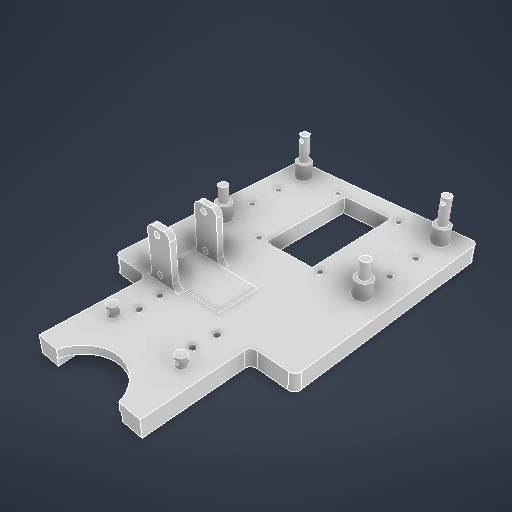
# Autodesk Inventor part: Lower_Chassis
Saved by Autodesk Inventor 2025 (Build 290162000, 162)
## iProperties
Created: 2024-06-03
Part Number: Lower_Chassis
Material: Generic
Document SubType Name: Modeling
Designer: Garfieldcmix
Density: 1 g/cm^3
Appearance: Default
Author: Garfieldcmix
Autodesk Inventor part; units mm, degrees
ref_plane "YZ Plane" through (0, 0, 0) normal (1, 0, 0) x (0, 1, 0)
ref_plane "XZ Plane" through (0, 0, 0) normal (0, 1, 0) x (-1, 0, 0)
derived "Car_Plan.ipt"
sketch "Car_Sketch" plane through (0, 0, 0) normal (0, 1, 0) x (-1, 0, 0)
  line L0 (0, 0) -> (94, 0)
  line L1 (0, 0) -> (0, 105)
  line L2 (94, 0) -> (94, 105)
  line L3 (0, 105) -> (20, 105)
  line L4 (20, 105) -> (20, 190)
  line L5 (20, 190) -> (74, 190)
  line L6 (74, 190) -> (74, 105)
  line L7 (74, 105) -> (94, 105)
  line L8 (-5, 68) -> (-5, 0)
  line L9 (-5, 0) -> (-32, 0)
  line L10 (-32, 0) -> (-32, 68)
  line L11 (-32, 68) -> (-5, 68)
  line L12 (47, 190) -> (47, 0) construction
  line L13 (126, 68) -> (99, 68)
  line L14 (99, 68) -> (99, 0)
  line L15 (126, 0) -> (126, 68)
  line L16 (99, 0) -> (126, 0)
  line L17 (-5, 34) -> (99, 34) construction
  line L18 (0, 95) -> (94, 95) construction
  line L19 (-5, 190) -> (-32, 190)
  line L20 (-32, 122) -> (-5, 122)
  line L21 (-32, 190) -> (-32, 122)
  line L22 (-5, 122) -> (-5, 190)
  line L23 (-5, 156) -> (99, 156) construction
  line L24 (126, 122) -> (99, 122)
  line L25 (126, 190) -> (126, 122)
  line L26 (99, 190) -> (126, 190)
  line L27 (99, 122) -> (99, 190)
  line L28 (0, 156) -> (47, 34) construction
  line L29 (94, 156) -> (47, 34) construction
  line L30 (0, 156) -> (-174.2341, 34) construction
  line L31 (-5, 34) -> (-174.2341, 34) construction
  line L32 (8.9873, 132.6713) -> (47, 142.55) construction
  line L33 (85.0127, 132.6713) -> (47, 142.55) construction
derived "Front_Bridge.ipt"
sketch "Front_Bridge_Base" plane through (0, 0, 0) normal (0, 1, 0) x (-1, 0, 0)
  circle A0 centre (0, 156) radius 1.5
  circle A1 centre (94, 156) radius 1.5
  line L0 (-5, 161) -> (-5, 151)
  line L1 (-5, 151) -> (29.5, 151)
  line L2 (99, 151) -> (99, 161)
  line L3 (99, 161) -> (90, 161)
  line L4 (4, 161) -> (22, 190)
  line L5 (22, 190) -> (72, 190)
  line L6 (72, 190) -> (90, 161)
  line L7 (0, 156) -> (94, 156) construction
  line L8 (4, 161) -> (-5, 161)
  line L9 (40.95, 172.3) -> (53.05, 172.3)
  line L10 (53.05, 172.3) -> (53.05, 149.9)
  line L11 (53.05, 149.9) -> (40.95, 149.9)
  line L12 (40.95, 149.9) -> (40.95, 172.3)
  line L13 (47, 156) -> (47, 149.9) construction
  line L14 (32, 151) -> (37, 144)
  line L15 (37, 144) -> (57, 144)
  line L16 (57, 144) -> (62, 151)
  line L17 (47, 156) -> (47, 144) construction
  line L18 (32, 151) -> (62, 151)
  line L19 (62, 151) -> (64.5, 151)
  line L20 (29.5, 151) -> (24.5, 102)
  line L21 (24.5, 102) -> (69.5, 102)
  line L22 (69.5, 102) -> (64.5, 151)
  line L23 (64.5, 151) -> (99, 151)
  line L24 (29.5, 151) -> (32, 151)
  line L25 (4, 161) -> (4, 151)
  line L26 (90, 161) -> (90, 151)
  circle A2 centre (32, 109) radius 1.5
  circle A3 centre (33, 119) radius 1.5
  line L27 (47, 156) -> (47, 102) construction
  circle A4 centre (61, 119) radius 1.5
  circle A5 centre (62, 109) radius 1.5
  line L28 (9, 169.0556) -> (9, 151)
  line L29 (84.8333, 151) -> (84.5992, 150.8961)
  line L30 (85, 169.0556) -> (85, 151)
  line L31 (26, 190) -> (26, 151)
  line L32 (68, 190) -> (68, 151)
  circle A6 centre (17, 157) radius 1.5
  circle A7 centre (17, 169) radius 1.5
  circle A8 centre (77, 157) radius 1.5
  circle A9 centre (77, 169) radius 1.5
  line L33 (37.95, 162.3) -> (33.95, 162.3)
  line L34 (33.95, 162.3) -> (33.95, 172.3)
  line L35 (33.95, 172.3) -> (37.95, 172.3)
  line L36 (37.95, 172.3) -> (37.95, 162.3)
  circle A10 centre (47, 156) radius 17.5
  line L37 (47, 156) -> (61.3352, 145.9624) construction
  line L38 (47, 156) -> (32.6648, 145.9624) construction
  line L39 (38.6848, 155.6711) -> (35.4082, 153.3768)
  line L40 (35.4082, 153.3768) -> (33.1139, 156.6535)
  line L41 (38.6848, 155.6711) -> (36.3905, 158.9478)
  line L42 (36.3905, 158.9478) -> (33.1139, 156.6535)
  line L43 (55.3152, 155.6711) -> (58.5918, 153.3768)
  line L44 (58.5918, 153.3768) -> (60.8861, 156.6535)
  line L45 (60.8861, 156.6535) -> (57.6095, 158.9478)
  line L46 (57.6095, 158.9478) -> (55.3152, 155.6711)
  line L47 (59.2478, 157.8006) -> (56.9535, 154.524) construction
  circle A11 centre (58.1006, 156.1623) radius 1.5
  line L48 (37.0465, 154.524) -> (34.7522, 157.8006) construction
  circle A12 centre (35.8994, 156.1623) radius 1.5
  point P0 (32.6648, 145.9624)
sketch "Chassis_Base" plane through (0, 0, 0) normal (0, 1, 0) x (-1, 0, 0)
  line L0 (29.5, 151) -> (24.5, 102) projected
  line L1 (-5, 151) -> (29.5, 151) projected
  line L2 (20, 105) -> (20, 190) projected
  line L3 (24.5, 102) -> (69.5, 102) projected
  line L4 (69.5, 102) -> (64.5, 151) projected
  circle A0 centre (61, 119) radius 1.5 projected
  circle A1 centre (62, 109) radius 1.5 projected
  circle A2 centre (33, 119) radius 1.5 projected
  circle A3 centre (32, 109) radius 1.5 projected
  line L5 (74, 190) -> (74, 105) projected
  line L6 (74, 105) -> (94, 105) projected
  line L7 (0, 105) -> (20, 105) projected
  line L8 (0, 0) -> (0, 105) projected
  line L9 (0, 0) -> (94, 0) projected
  line L10 (94, 0) -> (94, 105) projected
  line L11 (64.5, 151) -> (99, 151) projected
  line L12 (62, 151) -> (64.5, 151) projected
  line L13 (32, 151) -> (62, 151) projected
  line L14 (29.5, 151) -> (32, 151) projected
  line L15 (39.8, 103.8) -> (39.8, 100.8) construction
  line L16 (39.8, 79) -> (60.65, 79) construction
  line L17 (72.65, 79) -> (72.65, 82)
  line L18 (72.65, 103.8) -> (60.65, 103.8)
  line L19 (72.65, 100.8) -> (39.8, 100.8)
  line L20 (72.65, 82) -> (39.8, 82)
  line L21 (39.8, 100.8) -> (39.8, 82)
  line L22 (39.8, 82) -> (39.8, 79) construction
  line L23 (72.65, 100.8) -> (72.65, 103.8)
  line L24 (72.65, 82) -> (72.65, 100.8)
  line L25 (60.65, 103.8) -> (60.65, 100.8)
  line L26 (60.65, 82) -> (60.65, 79)
  line L27 (60.65, 103.8) -> (39.8, 103.8) construction
  line L28 (60.65, 79) -> (72.65, 79)
  line L29 (47, 190) -> (47, 0) construction
  circle A4 centre (29, 127) radius 2.4
  circle A5 centre (65, 127) radius 2.4
  circle A6 centre (47, 156) radius 17.5
  line L30 (-5, 156) -> (99, 156) construction
  point P0 (20, 151)
  point P1 (74, 151)
  point P2 (27.6351, 151)
  point P3 (66.3649, 151)
  point P4 (61.1421, 151)
  point P5 (32.8579, 151)
  point P6 (63.7705, 151)
  point P7 (30.2295, 151)
  point P8 (29.0999, 147.0789)
  point P9 (64.9001, 147.0789)
  dimension "d31" = 1.2
  dimension "d32" = 24.8
  dimension "d33" = 39.8
  dimension "d34" = 32.85
  dimension "d35" = 18.8
  dimension "d36" = 3
  dimension "d41" = 12
  dimension "d50" = 4.8
  dimension "d51" = 22
  dimension "d52" = 18
  dimension "d227" = 35
  constraints: 28 end point, 27 perpendicular, 4 point on line, 3 centre point, 3 vertical, 1 collinear, 1 midpoint, 1 symmetric about line, 1 other
  measures "d31" distance from line of L7 L15.start
  measures "d32" distance of L16.start L15.start
  measures "d33" distance from line of L8 L16.start
  measures "d34" distance of L17.start L16.start
  measures "d35" distance of L20.end L15.end
  measures "d36" distance between parallel lines of L19 L18
  measures "d41" distance between parallel lines of L23 L25
  measures "d50" diameter of A4
  measures "d51" distance from line of A4.centre L7
  measures "d52" distance from line of L29 A4.centre
  measures "d227" diameter of A6
extrude "Chassis_Base_Extrusion" add sketch "Chassis_Base" along normal blind 8 contours L14 A6 L12 L4 A5 L18 L25 L3 L0 A4 | L0 A4 L3 L25 L19 L21 L20 L26 L28 L17 L24 L23 L18 L4 A5 L11 L5 L6 L10 L9 L8 L7 L2 L1 | A4 L0 | L0 A4 | L14 L13 L12 A6 | L25 L18 L4 L3 | L3 L4 L18 L23 L19 L25 | A5 L4 | L4 A5 | L19 L24 L20 L21 | L17 L28 L26 L20 picked at (46.3222, 146.8728)
sketch "Lego_Frame_Connector" plane through (0, 8, 0) normal (0, 1, 0) x (1, 0, 0)
  line L0 (5, -34) -> (-99, -34) construction
  line L1 (0, -105) -> (0, 0) projected
  line L2 (-47, -190) -> (-47, 0) construction
  line L3 (-11.1, -10) -> (-11.1, -58) construction
  circle A0 centre (-11.1, -58) radius 3.9
  circle A1 centre (-11.1, -58) radius 2.4
  circle A2 centre (-11.1, -42) radius 1.5
  circle A3 centre (-11.1, -10) radius 3.9
  circle A4 centre (-11.1, -10) radius 2.4
  circle A5 centre (-11.1, -26) radius 1.5
  circle A6 centre (-82.9, -58) radius 3.9
  circle A7 centre (-82.9, -58) radius 2.4
  circle A8 centre (-82.9, -42) radius 1.5
  circle A9 centre (-82.9, -26) radius 1.5
  circle A10 centre (-82.9, -10) radius 3.9
  circle A11 centre (-82.9, -10) radius 2.4
  line L4 (-31, -10) -> (-31, -58) construction
  circle A12 centre (-31, -58) radius 1.5
  circle A13 centre (-31, -42) radius 1.5
  circle A14 centre (-31, -10) radius 1.5
  circle A15 centre (-31, -26) radius 1.5
  circle A16 centre (-63, -58) radius 1.5
  circle A17 centre (-63, -42) radius 1.5
  circle A18 centre (-63, -10) radius 1.5
  circle A19 centre (-63, -26) radius 1.5
  line L5 (-59.1, -58) -> (-34.9, -58)
  line L6 (-59.1, -58) -> (-59.1, -10)
  line L7 (-59.1, -10) -> (-34.9, -10)
  line L8 (-34.9, -10) -> (-34.9, -58)
  line L9 (-63, -10) -> (-59.1, -10) construction
  line L10 (-31, -10) -> (-34.9, -10) construction
  line L11 (-34.9, -58) -> (-31, -58) construction
  line L12 (-63, -58) -> (-59.1, -58) construction
  point P0 (-11.1, -34)
  point P1 (-31, -34)
  dimension "d237" = 7.8
  dimension "d238" = 4.8
  dimension "d239" = 35.9
  dimension "d240" = 3
  dimension "d242" = 16
  dimension "d243" = 8
  dimension "d245" = 16
  dimension "d246" = 3
  dimension "d248" = 3
  dimension "d252" = 16
  dimension "d253" = 8
  dimension "d325" = 24.2
  constraints: 20 centre point, 20 end point, 15 symmetric about line, 9 coincident, 4 point on line, 3 collinear, 3 horizontal, 2 midpoint, 2 perpendicular, 2 vertical, 15 other
  measures "d237" diameter of A0
  measures "d238" diameter of A1
  measures "d239" distance between parallel lines of L3 L2
  measures "d240" diameter of A2
  measures "d242" distance of L3.end point (-11.1, -42)
  measures "d243" distance from line of L0 point (-11.1, -42)
  measures "d245" distance between parallel lines of L4 L2
  measures "d246" diameter of A12
  measures "d248" diameter of A13
  measures "d252" distance of L4.end point (-31, -42)
  measures "d253" distance from line of L0 point (-31, -42)
  measures "d325" distance between parallel lines of L8 L6
extrude "Hole_For_Differential_Extrusion" cut sketch "Lego_Frame_Connector" against normal up to surface (8 mm away) contours L6 L7 L8 L5
extrude "Lego_Frame_Connector_Extrusion" add sketch "Lego_Frame_Connector" along normal blind 8 contours A0 | A1 | A3 | A4 | A6 | A7 | A10 | A11
extrude "Lego_Frame_Connector_2_Extrusion" add sketch "Lego_Frame_Connector" along normal blind 8 from surface at 8 contours A1 | A4 | A7 | A11
extrude "Extrusion24" cut sketch "Lego_Frame_Connector" against normal through all contours A2 | A5 | A8 | A9 | A12 | A14 | A16 | A18
extrude "Extrusion23" cut sketch "Lego_Frame_Connector" against normal blind 7 contours A1 | A4 | A7 | A11
extrude "Motor_Base_Extrusion" add sketch "Chassis_Base" along normal blind 8.75 contours L19 L24 L20 L21
extrude "Motor_Holder_Extrusion" add sketch "Chassis_Base" along normal blind 32 contours L25 L18 L4 L3 | L3 L4 L18 L23 L19 L25 | L17 L28 L26 L20
sketch "Motor_Screw_Hole" plane through (-60.65, 8, 79) normal (0, 0, -1) x (-1, 0, 0)
  circle A0 centre (6.95, 3.25) radius 1.5
  circle A1 centre (6.95, 20.75) radius 1.5
  line L0 (12, 0) -> (0, 0) projected
  line L1 (12, 0) -> (12, 24) projected
  point P0 (-60.65, -8)
  dimension "d42" = 3
  dimension "d43" = 3
  dimension "d44" = 3.25
  dimension "d45" = 5.05
  dimension "d46" = 17.5
  dimension "d47" = 5.05
  constraints: 2 centre point
  measures "d42" diameter of A0
  measures "d43" diameter of A1
  measures "d44" distance from line of L0 A0.centre
  measures "d45" distance from line of L1 A0.centre
  measures "d46" distance of A1.centre A0.centre
  measures "d47" distance from line of L1 A1.centre
extrude "Motor_Screw_Hole_Extrusion" cut sketch "Motor_Screw_Hole" against normal through all
extrude "Front_Bridge_Connector_Extrusion" cut sketch "Chassis_Base" along normal blind 4 contours L14 A6 L12 L4 A5 L18 L25 L3 L0 A4 | A4 L0 | L14 L13 L12 A6 | L25 L18 L4 L3 | L4 A5 picked at (28.4588, 127.787) picked at (46.3222, 146.8728) picked at (64.2025, 126.8439)
extrude "Extrusion17" cut sketch "Chassis_Base" along normal blind 10 contours L14 L13 L12 A6 picked at (46.3222, 146.8728)
sketch "1.5_Base_Screw" plane through (0, 8, 0) normal (0, 1, 0) x (1, 0, 0)
  circle A0 centre (-29, -127) radius 2.4 projected
  circle A1 centre (-65, -127) radius 2.4 projected
  point P0 (0, 0)
extrude "Extrusion22" cut sketch "1.5_Base_Screw" against normal blind 3
offset faces "Size8" outward 1.6 faces at (-67.0285, 6, 128.2827) (-31.0285, 6, 128.2827)
extrude "Pillar_Foundation_Extrusion" add sketch "1.5_Base_Screw" along normal blind 5
ref_plane "Foundation_Hole_Work_Plane" through (-29, 8, 129.4) normal (0, 0, 1) x (1, 0, 0)
sketch "Foundation_Hole_Sketch" plane through (-29, 8, 129.4) normal (0, 0, 1) x (1, 0, 0)
  line L0 (-33.6, 5) -> (-38.4, 5) construction
  line L1 (2.4, 5) -> (-2.4, 5) construction
  line L2 (-36, 5) -> (-36, 2.5) construction
  line L3 (0, 5) -> (0, 2.5) construction
  dimension "d208" = 2.5
  dimension "d209" = 2.5
  constraints: 4 end point, 2 midpoint, 2 perpendicular
  measures "d208" distance of L2.end L2.start
  measures "d209" distance of L3.end L3.start
hole "Foundation_Hole" at (-65, 10.5, 129.4) at (-29, 10.5, 129.4) direction (0, 0, -1) diameter 2 depth 4.8 tip angle 118
extrude "Pillar_Foundation_2_Extrusion" add sketch "Lego_Frame_Connector" along normal blind 21 contours A4 | A11
ref_plane "Foundation_2_Hole_Work_Plane" through (-11.1, 8, 12.4) normal (0, 0, 1) x (1, 0, 0)
sketch "Foundation_3_Hole_Sketch" plane through (-11.1, 8, 12.4) normal (0, 0, 1) x (1, 0, 0)
  line L0 (2.4, 21) -> (-2.4, 21) projected
  line L1 (-69.4, 21) -> (-74.2, 21) projected
  line L2 (0, 21) -> (0, 18.5) construction
  line L3 (-71.8, 21) -> (-71.8, 18.5) construction
  point P0 (11.1, -8)
  dimension "d254" = 2.5
  dimension "d255" = 2.5
  constraints: 4 end point, 2 coincident, 2 midpoint, 2 perpendicular
  measures "d254" distance of L2.start L2.end
  measures "d255" distance of L3.start L3.end
hole "Foundation_3_Hole" at (-11.1, 26.5, 12.4) at (-82.9, 26.5, 12.4) direction (0, 0, -1) diameter 2 depth 4.8 tip angle 118
fillet "Fillet1" radius 3 6 edges at (-20, 4, 105) (0, 4, 105) (0, 4, 0) (-94, 4, 0) (-94, 4, 105) (-74, 4, 105)
fillet "Fillet2" radius 3 7 edges at (-72.65, 32, 102.3) (-60.65, 32, 102.3) (-60.65, 32, 80.5) (-72.65, 32, 80.5) (-60.65, 8, 102.3) (-72.65, 8, 91.4) (-60.65, 8, 80.5)
offset faces "Size1" outward -0.1 faces at (-62.6826, 17.4948, 100.8) (-62.6826, 22.5052, 82)
offset faces "Size7" outward -0.13 faces at (-66.9187, 11.3333, 128.4418) (-30.9187, 11.3333, 128.4418) (-80.5078, 24.6667, 10.1931) (-8.7078, 24.6667, 10.1931) (-8.7078, 21.3333, 58.1931) (-80.5078, 21.3333, 58.1931)
body "Solid1"
